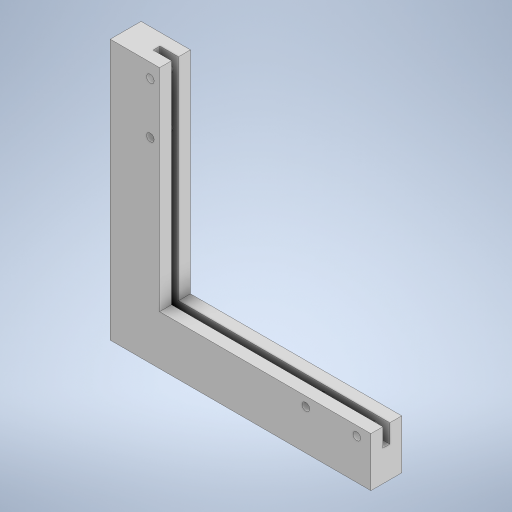
# Autodesk Inventor part: UCD V1.0 PCB Holder
Saved by Autodesk Inventor 2024 (Build 280153000, 153)
## iProperties
Created: 2024-10-24
Part Number: UCD V1.0 PCB Holder
Material: Generic
Document SubType Name: Modeling
Designer: Kemper Room 121
Density: 1 g/cm^3
Appearance: Default
Author: Kemper Room 121
Autodesk Inventor part; units mm, degrees
ref_plane "YZ Plane" through (0, 0, 0) normal (1, 0, 0) x (0, 1, 0)
ref_plane "XZ Plane" through (0, 0, 0) normal (0, 1, 0) x (-1, 0, 0)
ref_plane "XY Plane" through (0, 0, 0) normal (0, 0, 1) x (1, 0, 0)
sketch "Sketch1" plane through (0, 0, 0) normal (0, 0, 1) x (1, 0, 0)
  line L0 (0, 0) -> (0, 10)
  line L1 (0, 10) -> (0, 78.5)
  line L2 (0, 78.5) -> (0, 84.5)
  line L3 (0, 84.5) -> (10, 84.5)
  line L4 (10, 84.5) -> (16, 84.5)
  line L5 (16, 84.5) -> (16, 16)
  line L6 (16, 16) -> (84.5, 16)
  line L7 (84.5, 0) -> (0, 0)
  line L8 (10, 84.5) -> (10, 10)
  line L9 (84.5, 16) -> (84.5, 10)
  line L10 (84.5, 10) -> (84.5, 0)
  line L11 (84.5, 0) -> (0, 0)
  line L12 (84.5, 10) -> (10, 10)
  circle A0 centre (13, 79.9) radius 1.25
  circle A1 centre (13, 63.4) radius 1.25
  line L13 (13, 82.5899) -> (13, 13)
  circle A2 centre (63.4, 13) radius 1.25
  circle A3 centre (79.9, 13) radius 1.25
  point P0 (13, 84.5)
  dimension "d0" = 68.5
  dimension "d1" = 10
  dimension "d2" = 10
  dimension "d3" = 6
  dimension "d6" = 10
  dimension "d7" = 6
  dimension "d8" = 0
  dimension "d9" = 2.5
  dimension "d11" = 6
  dimension "d13" = 69.9
  dimension "d14" = 2.5
  dimension "d15" = 53.4
  dimension "d16" = 0
  dimension "d17" = 84.5
  dimension "d20" = 90
  constraints: 28 end point, 4 centre point, 4 perpendicular, 3 parallel, 3 point on line, 2 vertical, 1 collinear, 1 horizontal, 1 midpoint, 5 other
  measures "d0" distance of L0.end L1.end
  measures "d1" distance of L0.start L0.end
  measures "d2" distance of L2.end L3.end
  measures "d3" distance of L3.end L4.end
  measures "d6" distance of L9.end L7.start
  measures "d7" distance of L6.end L9.end
  measures "d8" horizontal distance of A0.centre point (13, 84.5)
  measures "d9" diameter of A0
  measures "d11" distance of L1.end L2.end
  measures "d13" distance from line of L12 A0.centre
  measures "d14" diameter of A1
  measures "d15" distance from line of L12 A1.centre
  measures "d16" horizontal distance of point (13, 84.5) A1.centre
  measures "d17" distance of L7.start L0.start
extrude "Extrusion1" add sketch "Sketch1" along normal blind 3.875
sketch "Sketch2" plane through (0, 0, 3.875) normal (0, 0, 1) x (1, 0, 0)
  line L0 (0, 0) -> (84.5, 0) projected
  line L1 (84.5, 0) -> (84.5, 16) projected
  line L2 (84.5, 16) -> (16, 16) projected
  line L3 (16, 16) -> (16, 84.5) projected
  line L4 (16, 84.5) -> (0, 84.5) projected
  line L5 (0, 84.5) -> (0, 0) projected
  circle A0 centre (13, 63.4) radius 1.25 projected
  circle A1 centre (13, 79.9) radius 1.25 projected
  circle A2 centre (63.4, 13) radius 1.25 projected
  circle A3 centre (79.9, 13) radius 1.25 projected
  line L6 (0, 0) -> (5.4402, 0)
  line L7 (10, 10) -> (10, 84.5)
  line L8 (10, 84.5) -> (0, 84.5)
  line L9 (0, 84.5) -> (0, 0)
  line L10 (84.5, 0) -> (84.5, 16) projected
  line L11 (0, 0) -> (84.5, 0)
  line L12 (84.5, 0) -> (84.5, 10)
  line L13 (84.5, 10) -> (10, 10)
  line L14 (0, 5.0322) -> (0, 0)
  dimension "d24" = 10
  dimension "d25" = 10
  constraints: 16 end point, 4 parallel, 2 horizontal, 2 perpendicular, 2 point on line
  measures "d24" distance of L7.end L4.end
  measures "d25" distance between parallel lines of L11 L13
extrude "Extrusion2" add sketch "Sketch2" along normal blind 2.25 contours L5 L4 L7 L13 L1 L0
sketch "Sketch5" plane through (0, 0, 6.125) normal (0, 0, 1) x (1, 0, 0)
  line L0 (10, 10) -> (10, 84.5) projected
  line L1 (10, 84.5) -> (0, 84.5) projected
  line L2 (0, 84.5) -> (0, 0) projected
  line L3 (0, 0) -> (84.5, 0) projected
  line L4 (84.5, 0) -> (84.5, 10) projected
  line L5 (84.5, 10) -> (10, 10) projected
  circle A0 centre (79.9, 13) radius 1.25 projected
  circle A1 centre (63.4, 13) radius 1.25 projected
  circle A2 centre (13, 79.9) radius 1.25 projected
  circle A3 centre (13, 63.4) radius 1.25 projected
  line L6 (10, 84.5) -> (10, 10) projected
  line L7 (10, 10) -> (84.5, 10) projected
  line L8 (84.5, 10) -> (84.5, 16) projected
  line L9 (84.5, 16) -> (16, 16) projected
  line L10 (16, 16) -> (16, 84.5) projected
  line L11 (16, 84.5) -> (10, 84.5) projected
  line L12 (0, 84.5) -> (16, 84.5)
  line L13 (16, 0) -> (0, 0)
  line L14 (0, 0) -> (0, 84.5)
  line L15 (0, 0) -> (84.5, 0)
  line L16 (84.5, 0) -> (84.5, 16)
  line L17 (84.5, 16) -> (16, 16)
  line L18 (0, 16) -> (0, 0)
  line L19 (16, 84.5) -> (16, 16)
  constraints: 17 end point, 4 parallel, 2 horizontal, 2 perpendicular, 1 point on line
extrude "Extrusion5" add sketch "Sketch5" along normal blind 3.875 contours L5 L4 L3 L2 L1 L0 | L0 L11 L10 L9 L8 L5 | A0 | A1 | A2 | A3
sketch "Sketch6" plane through (0, 0, 0) normal (-1, 0, 0) x (0, 0, 1)
  line L0 (3.875, 84.5) -> (3.875, 10) projected
  line L1 (3.875, 84.5) -> (6.125, 84.5) projected
  line L2 (6.125, 10) -> (6.125, 84.5) projected
  line L3 (3.875, 10) -> (6.125, 10) projected
  line L4 (0, 84.5) -> (10, 84.5) projected
  line L5 (0, 84.5) -> (0, 0) projected
  line L6 (0, 0) -> (10, 0) projected
  line L7 (10, 84.5) -> (10, 0) projected
  circle A0 centre (5, 44.25) radius 2
  circle A1 centre (5, 34) radius 2
  point P0 (6.125, 47.25)
  dimension "d51" = 4
  dimension "d52" = 4
  dimension "d53" = 10
  dimension "d54" = 5
  dimension "d55" = 5
  dimension "d73" = 24
  dimension "d74" = 34.25
  constraints: 2 centre point, 1 midpoint
  measures "d51" diameter of A0
  measures "d52" diameter of A1
  measures "d53" distance of L4.start L4.end
  measures "d54" distance from line of L5 A1.centre
  measures "d55" distance from line of L5 A0.centre
  measures "d73" distance from line of L3 A1.centre
  measures "d74" distance from line of L3 A0.centre
extrude "Extrusion6" cut sketch "Sketch6" against normal blind 10 contours A0 L2 L0 | L0 A0 | A0 L2 | A1 L2 L0 | L0 A1 | A1 L2
sketch "Sketch7" plane through (0, 0, 0) normal (0, -1, 0) x (1, 0, 0)
  line L0 (10, 3.875) -> (84.5, 3.875) projected
  line L1 (10, 3.875) -> (10, 6.125) projected
  line L2 (84.5, 6.125) -> (10, 6.125) projected
  line L3 (84.5, 3.875) -> (84.5, 6.125) projected
  line L4 (0, 0) -> (0, 10) projected
  line L5 (0, 0) -> (84.5, 0) projected
  line L6 (84.5, 0) -> (84.5, 10) projected
  line L7 (0, 10) -> (84.5, 10) projected
  circle A0 centre (44.25, 5) radius 2
  circle A1 centre (38, 5) radius 2
  point P0 (84.5, 5)
  dimension "d60" = 4
  dimension "d61" = 4
  dimension "d62" = 10
  dimension "d63" = 5
  dimension "d64" = 5
  dimension "d77" = 28
  dimension "d78" = 34.25
  constraints: 2 centre point, 1 midpoint
  measures "d60" diameter of A0
  measures "d61" diameter of A1
  measures "d62" distance of L5.end L6.end
  measures "d63" distance from line of L5 A1.centre
  measures "d64" distance from line of L5 A0.centre
  measures "d77" distance from line of L1 A1.centre
  measures "d78" distance from line of L1 A0.centre
extrude "Extrusion7" cut sketch "Sketch7" against normal blind 10 contours A1 L2 L0 | L0 A1 | A1 L2 | A0 L2 L0 | L0 A0 | A0 L2
sketch "Sketch8" plane through (0, 0, 0) normal (0, 0, -1) x (-1, 0, 0)
  line L0 (0, 0) -> (-84.5, 0) projected
  line L1 (0, 84.5) -> (0, 0) projected
  line L2 (-16, 84.5) -> (0, 84.5) projected
  line L3 (-16, 16) -> (-16, 84.5) projected
  line L4 (-84.5, 16) -> (-16, 16) projected
  line L5 (-84.5, 0) -> (-84.5, 16) projected
  circle A0 centre (-13, 63.4) radius 1.25 projected
  circle A1 centre (-13, 79.9) radius 1.25 projected
  circle A2 centre (-63.4, 13) radius 1.25 projected
  circle A3 centre (-79.9, 13) radius 1.25 projected
  circle A4 centre (-79.9, 13) radius 1.25
  circle A5 centre (-63.4, 13) radius 1.25
  circle A6 centre (-13, 63.4) radius 1.25
  circle A7 centre (-13, 79.9) radius 1.25
  constraints: 4 centre point, 4 coincident, 4 concentric
extrude "Extrusion8" cut sketch "Sketch8" against normal through all contours A0 | A1 | A2 | A3
equation "\"d0\" = PCB_L"
equation "\"d1\" = Clamp_Bracket_W"
equation "\"d2\" = Clamp_Bracket_W"
equation "\"d3\" = Trim_Mount_W"
equation "\"d6\" = d1"
equation "\"d7\" = d3"
equation "\"d11\" = Trim_Mount_W"
equation "\"d14\" = d9"
equation "\"d17\" = d0 + d1 + d11"
equation "\"d22\" = Mount_W_Back"
equation "\"d24\" = Clamp_Bracket_W"
equation "\"d25\" = Clamp_Bracket_W"
equation "\"d49\" = Mount_W_Front"
equation "\"d51\" = Post_Mount_Hole_D"
equation "\"d52\" = d51"
equation "\"d54\" = 0.5 * d53"
equation "\"d55\" = 0.5 * d53"
equation "\"d73\" = 0.5 * PCB_W - PCB_W_Offset"
equation "\"d74\" = 0.5 * PCB_L"
equation "\"d58\" = Clamp_Bracket_W"
equation "\"d60\" = d51"
equation "\"d61\" = d51"
equation "\"d63\" = 0.5 * d62"
equation "\"d64\" = 0.5 * d62"
equation "\"d77\" = 0.5 * PCB_W + PCB_W_Offset"
equation "\"d78\" = 0.5 * PCB_L"
equation "\"d67\" = Clamp_Bracket_W"
equation "\"PCB_L\" = 68.5"
equation "\"Clamp_Bracket_W\" = 10"
equation "\"Trim_Mount_W\" = 6"
equation "\"Mount_W_Back\" = 3.875"
equation "\"Mount_W_Front\" = 3.875"
equation "\"Post_Mount_Hole_D\" = 4"
equation "\"PCB_W\" = 52"
equation "\"PCB_W_Offset\" = 2"
body "Solid1"
